Autodesk Fusion 360 part; units mm, degrees
(part 2 of 2)
sketch "Sketch6" plane through (0, 0, -2) normal (0, 0, -1) x (1, 0, 0)
  spline S0 degree 3 poles (37.9249, 4.0377) (34.348, 1.7603) (29.402, 0.3264) (25.1373, 0.3305) knots 0 0 0 0 1 1 1 1
  spline S1 degree 3 poles (25.1373, 0.3305) (25.0915, 0.3305) (25.0457, 0.3307) (25, 0.3309) knots 0 0 0 0 0.011443 0.011443 0.011443 0.011443
  spline S2 degree 3 poles (25, 0.3309) (24.9543, 0.3307) (24.9085, 0.3305) (24.8627, 0.3305) knots -0.011443 -0.011443 -0.011443 -0.011443 0 0 0 0
  spline S3 degree 3 poles (24.8627, 0.3305) (20.598, 0.3264) (15.652, 1.7603) (12.0751, 4.0377) knots -1 -1 -1 -1 0 0 0 0
  spline S4 degree 3 poles (12.0751, 4.0377) (9.8012, 5.4854) (7.8971, 7.1098) (6.2927, 8.9882) knots -1 -1 -1 -1 -0.448955 -0.448955 -0.448955 -0.448955
  spline S5 degree 5 poles (6.2927, 8.9882) (6.7312, 9.5928) (7.5942, 10.7006) (8.8467, 12.0587) (10.4463, 13.3414) (12.3768, 14.3264) (13.9094, 14.7689) (15.0688, 14.9371) (15.8476, 14.9755) (16.2364, 14.9764) knots 0 0 0 0 0 0 0.2 0.4 0.6 0.8 0.997509 0.997509 0.997509 0.997509 0.997509 0.997509
  spline S6 degree 3 poles (16.2364, 14.9764) (16.2539, 14.4812) (16.2926, 14.0359) (16.3533, 13.7321) knots 0.672801 0.672801 0.672801 0.672801 1 1 1 1
  spline S7 degree 3 poles (16.3533, 13.7321) (16.7289, 11.8523) (17.4711, 10.4695) (18.4214, 9.8792) knots 0 0 0 0 1 1 1 1
  spline S8 degree 3 poles (18.4214, 9.8792) (18.7703, 9.6625) (18.8263, 9.6487) (19.3578, 9.6487) knots 0 0 0 0 1 1 1 1
  spline S9 degree 3 poles (19.3578, 9.6487) (19.8618, 9.6487) (19.958, 9.6692) (20.2453, 9.8381) knots 0 0 0 0 1 1 1 1
  spline S10 degree 3 poles (20.2453, 9.8381) (21.4794, 10.5634) (22.3435, 12.632) (22.4858, 14.9765) knots 0 0 0 0 0.816867 0.816867 0.816867 0.816867
  line L0 (22.4858, 14.9765) -> (27.5142, 14.9765)
  spline S11 degree 3 poles (27.5142, 14.9765) (27.6565, 12.632) (28.5206, 10.5634) (29.7547, 9.8381) knots -0.816867 -0.816867 -0.816867 -0.816867 0 0 0 0
  spline S12 degree 3 poles (29.7547, 9.8381) (30.042, 9.6692) (30.1382, 9.6487) (30.6422, 9.6487) knots -1 -1 -1 -1 0 0 0 0
  spline S13 degree 3 poles (30.6422, 9.6487) (31.1737, 9.6487) (31.2297, 9.6625) (31.5786, 9.8792) knots -1 -1 -1 -1 0 0 0 0
  spline S14 degree 3 poles (31.5786, 9.8792) (32.5289, 10.4695) (33.2711, 11.8523) (33.6467, 13.7321) knots -1 -1 -1 -1 0 0 0 0
  spline S15 degree 3 poles (33.6467, 13.7321) (33.7074, 14.0359) (33.7461, 14.4812) (33.7636, 14.9764) knots -1 -1 -1 -1 -0.672801 -0.672801 -0.672801 -0.672801
  spline S16 degree 5 poles (33.7636, 14.9764) (34.1524, 14.9755) (34.9312, 14.9371) (36.0906, 14.7689) (37.6232, 14.3264) (39.5537, 13.3414) (41.1533, 12.0587) (42.4058, 10.7006) (43.2688, 9.5928) (43.7073, 8.9882) knots -0.997509 -0.997509 -0.997509 -0.997509 -0.997509 -0.997509 -0.8 -0.6 -0.4 -0.2 0 0 0 0 0 0
  spline S17 degree 3 poles (43.7073, 8.9882) (42.1029, 7.1098) (40.1988, 5.4854) (37.9249, 4.0377) knots 0.448955 0.448955 0.448955 0.448955 1 1 1 1
  line L1 (26, 42.9197) -> (26, 49.8323)
  spline S18 degree 3 poles (26, 49.8323) (26.5653, 49.8125) (27.1076, 49.7746) (27.6071, 49.7183) knots 0.743062 0.743062 0.743062 0.743062 1 1 1 1
  spline S19 degree 3 poles (27.6071, 49.7183) (31.8916, 49.2352) (35.9396, 47.6727) (39.3823, 45.1732) knots 0 0 0 0 1 1 1 1
  spline S20 degree 3 poles (39.3823, 45.1732) (40.6259, 44.2703) (41.223, 43.7559) (42.4276, 42.5496) knots 0 0 0 0 1 1 1 1
  spline S21 degree 3 poles (42.4276, 42.5496) (44.1166, 40.8584) (45.373, 39.2036) (46.5306, 37.1458) knots 0 0 0 0 1 1 1 1
  spline S22 degree 3 poles (46.5306, 37.1458) (47.3561, 35.6786) (48.2602, 33.529) (48.6498, 32.1074) knots 0 0 0 0 1 1 1 1
  spline S23 degree 3 poles (48.6498, 32.1074) (48.7491, 31.7452) (48.8843, 31.2562) (48.9503, 31.0207) knots 0 0 0 0 1 1 1 1
  spline S24 degree 3 poles (48.9503, 31.0207) (49.1719, 30.2294) (49.3568, 29.1578) (49.4818, 28.0278) knots 0 0 0 0 0.470145 0.470145 0.470145 0.470145
  spline S25 degree 3 poles (49.4818, 28.0278) (47.9315, 28.8817) (46.4271, 29.3185) (45.0223, 29.384) (43.136, 29.4719) (41.4621, 28.9779) (40.0154, 28.0751) knots 0.091067 0.091067 0.091067 0.091067 0.417024 0.417024 0.417024 0.85471 0.85471 0.85471 0.85471
  spline S26 degree 3 poles (40.0154, 28.0751) (40.0053, 28.8306) (39.9736, 29.2565) (39.904, 29.7035) knots -0.761621 -0.761621 -0.761621 -0.761621 0 0 0 0
  spline S27 degree 3 poles (39.904, 29.7035) (39.3804, 33.0647) (37.9288, 36.0367) (35.6546, 38.4035) knots -1 -1 -1 -1 0 0 0 0
  spline S28 degree 3 poles (35.6546, 38.4035) (34.8864, 39.2029) (33.7866, 40.1121) (32.9419, 40.646) knots -1 -1 -1 -1 0 0 0 0
  spline S29 degree 3 poles (32.9419, 40.646) (31.0907, 41.8162) (28.4901, 42.7183) (26.4545, 42.8964) knots -1 -1 -1 -1 0 0 0 0
  spline S30 degree 3 poles (26.4545, 42.8964) (26.3388, 42.9066) (26.1819, 42.9143) (26, 42.9197) knots -1 -1 -1 -1 -0.809548 -0.809548 -0.809548 -0.809548
  spline S31 degree 3 poles (24, 42.9197) (23.8181, 42.9143) (23.6612, 42.9066) (23.5455, 42.8964) knots 0.809548 0.809548 0.809548 0.809548 1 1 1 1
  spline S32 degree 3 poles (23.5455, 42.8964) (21.5099, 42.7183) (18.9093, 41.8162) (17.0581, 40.646) knots 0 0 0 0 1 1 1 1
  spline S33 degree 3 poles (17.0581, 40.646) (16.2134, 40.1121) (15.1136, 39.2029) (14.3454, 38.4035) knots 0 0 0 0 1 1 1 1
  spline S34 degree 3 poles (14.3454, 38.4035) (12.0712, 36.0367) (10.6196, 33.0647) (10.096, 29.7035) knots 0 0 0 0 1 1 1 1
  spline S35 degree 3 poles (10.096, 29.7035) (10.0264, 29.2565) (9.9947, 28.8306) (9.9846, 28.0751) knots 0 0 0 0 0.761621 0.761621 0.761621 0.761621
  spline S36 degree 3 poles (9.9846, 28.0751) (8.5379, 28.9779) (6.864, 29.4719) (4.9777, 29.384) (3.5729, 29.3185) (2.0685, 28.8817) (0.5182, 28.0278) knots -0.85471 -0.85471 -0.85471 -0.85471 -0.417024 -0.417024 -0.417024 -0.091067 -0.091067 -0.091067 -0.091067
  spline S37 degree 3 poles (0.5182, 28.0278) (0.6432, 29.1578) (0.8281, 30.2294) (1.0497, 31.0207) knots -0.470145 -0.470145 -0.470145 -0.470145 0 0 0 0
  spline S38 degree 3 poles (1.0497, 31.0207) (1.1157, 31.2562) (1.2509, 31.7452) (1.3502, 32.1074) knots -1 -1 -1 -1 0 0 0 0
  spline S39 degree 3 poles (1.3502, 32.1074) (1.7398, 33.529) (2.6439, 35.6786) (3.4694, 37.1458) knots -1 -1 -1 -1 0 0 0 0
  spline S40 degree 3 poles (3.4694, 37.1458) (4.627, 39.2036) (5.8834, 40.8584) (7.5724, 42.5496) knots -1 -1 -1 -1 0 0 0 0
  spline S41 degree 3 poles (7.5724, 42.5496) (8.777, 43.7559) (9.3741, 44.2703) (10.6177, 45.1732) knots -1 -1 -1 -1 0 0 0 0
  spline S42 degree 3 poles (10.6177, 45.1732) (14.0604, 47.6727) (18.1084, 49.2352) (22.3929, 49.7183) knots -1 -1 -1 -1 0 0 0 0
  spline S43 degree 3 poles (22.3929, 49.7183) (22.8924, 49.7746) (23.4347, 49.8125) (24, 49.8323) knots -1 -1 -1 -1 -0.743062 -0.743062 -0.743062 -0.743062
  line L2 (24, 49.8323) -> (24, 42.9197)
  spline S44 degree 3 poles (49.6438, 24.3029) (49.4952, 20.5588) (48.6987, 17.4096) (47.0703, 14.1273) knots 0 0 0 0 1 1 1 1
  spline S45 degree 3 poles (47.0703, 14.1273) (46.493, 12.9638) (45.8561, 11.8785) (45.1508, 10.8618) knots 0 0 0 0 0.273539 0.273539 0.273539 0.273539
  spline S46 degree 3 poles (45.1508, 10.8618) (43.4717, 13.1181) (41.7533, 14.5837) (40.0547, 15.4812) (38.2296, 16.4456) (36.4871, 16.8223) (34.777, 16.9413) (34.4324, 16.9653) (34.0883, 16.9769) (33.7445, 16.9765) (33.738, 16.9765) (33.7315, 16.9765) (33.725, 16.9765) knots 0.013228 0.013228 0.013228 0.013228 0.443948 0.443948 0.443948 0.906729 0.906729 0.906729 1 1 1 1.00195 1.00195 1.00195 1.00195
  ellipse E0 centre (33.3549, 15.0887) end of major axis (33.411, 18.2873) minor radius 0.4181 (33.725, 16.9765) -> (33.6101, 17.8664) ccw
  spline S47 degree 3 poles (33.6101, 17.8664) (33.169, 19.9501) (32.2562, 21.4052) (31.1636, 21.7662) knots -1 -1 -1 -1 0 0 0 0
  spline S48 degree 3 poles (31.1636, 21.7662) (30.3753, 22.0267) (29.4073, 21.5865) (28.8005, 20.6915) knots -1 -1 -1 -1 0 0 0 0
  spline S49 degree 3 poles (28.8005, 20.6915) (28.1198, 19.6876) (27.7379, 18.5421) (27.5687, 16.9765) knots -1 -1 -1 -1 -0.075763 -0.075763 -0.075763 -0.075763
  line L3 (27.5687, 16.9765) -> (22.4313, 16.9765)
  spline S50 degree 3 poles (22.4313, 16.9765) (22.2621, 18.5421) (21.8802, 19.6876) (21.1995, 20.6915) knots 0.075763 0.075763 0.075763 0.075763 1 1 1 1
  spline S51 degree 3 poles (21.1995, 20.6915) (20.5927, 21.5865) (19.6247, 22.0267) (18.8364, 21.7662) knots 0 0 0 0 1 1 1 1
  spline S52 degree 3 poles (18.8364, 21.7662) (17.7438, 21.4052) (16.831, 19.9501) (16.3899, 17.8664) knots 0 0 0 0 1 1 1 1
  ellipse E1 centre (16.6451, 15.0887) end of major axis (16.7011, 11.8901) minor radius 0.4181 (16.3899, 17.8664) -> (16.275, 16.9765) ccw
  spline S53 degree 3 poles (16.275, 16.9765) (16.2685, 16.9765) (16.262, 16.9765) (16.2555, 16.9765) (15.9117, 16.9769) (15.5676, 16.9653) (15.223, 16.9413) (13.5129, 16.8223) (11.7704, 16.4456) (9.9453, 15.4812) (8.2467, 14.5837) (6.5283, 13.1181) (4.8492, 10.8618) knots -1.00195 -1.00195 -1.00195 -1.00195 -1 -1 -1 -0.906729 -0.906729 -0.906729 -0.443948 -0.443948 -0.443948 -0.013228 -0.013228 -0.013228 -0.013228
  spline S54 degree 3 poles (4.8492, 10.8618) (4.1439, 11.8785) (3.507, 12.9638) (2.9297, 14.1273) knots -0.273539 -0.273539 -0.273539 -0.273539 0 0 0 0
  spline S55 degree 3 poles (2.9297, 14.1273) (1.3013, 17.4096) (0.5048, 20.5588) (0.3562, 24.3029) knots -1 -1 -1 -1 0 0 0 0
  ellipse E2 centre (1.5341, 27.8391) end of major axis (0.9284, 22.1103) minor radius 1.0317 (0.3495, 25.5702) -> (0.3562, 24.3029) ccw
  spline S56 degree 5 poles (0.3495, 25.5702) (0.8642, 25.9274) (1.8614, 26.5452) (3.261, 27.1829) (4.9563, 27.5281) (6.8533, 27.3542) (8.214, 26.8513) (9.1392, 26.2868) (9.7099, 25.8236) (9.9837, 25.5702) knots 0 0 0 0 0 0 0.2 0.4 0.6 0.8 1 1 1 1 1 1
  line L4 (9.9837, 25.5702) -> (9.5685, 25.3593)
  spline S57 degree 3 poles (9.5685, 25.3593) (8.985, 25.0629) (8.7925, 24.7926) (8.7925, 24.2699) knots 0 0 0 0 1 1 1 1
  spline S58 degree 3 poles (8.7925, 24.2699) (8.7925, 23.9246) (8.8206, 23.8276) (8.9823, 23.6157) knots 0 0 0 0 1 1 1 1
  spline S59 degree 3 poles (8.9823, 23.6157) (9.0867, 23.4788) (9.271, 23.3255) (9.3918, 23.275) knots 0 0 0 0 1 1 1 1
  spline S60 degree 3 poles (9.3918, 23.275) (9.865, 23.0773) (10.0223, 23.1273) (11.92, 24.0791) knots 0 0 0 0 1 1 1 1
  spline S61 degree 3 poles (11.92, 24.0791) (13.4801, 24.8616) (13.727, 25.0063) (13.87, 25.2225) knots 0 0 0 0 1 1 1 1
  spline S62 degree 3 poles (13.87, 25.2225) (14.3541, 25.9539) (13.9374, 26.8519) (13.081, 26.923) knots 0 0 0 0 1 1 1 1
  spline S63 degree 3 poles (13.081, 26.923) (12.7923, 26.9469) (12.6703, 26.9186) (12.3363, 26.7499) knots 0 0 0 0 1 1 1 1
  ellipse E3 centre (12.2838, 26.7829) end of major axis (12.6728, 26.975) minor radius 0.053 (11.8959, 26.5891) -> (12.3363, 26.7499) ccw
  spline S64 degree 3 poles (11.8959, 26.5891) (11.7452, 26.7398) (11.9635, 29.5037) (12.2147, 30.6256) knots 0 0 0 0 1 1 1 1
  spline S65 degree 3 poles (12.2147, 30.6256) (12.3647, 31.2958) (12.9496, 32.9532) (13.2453, 33.5457) knots 0 0 0 0 1 1 1 1
  spline S66 degree 3 poles (13.2453, 33.5457) (14.0979, 35.2549) (15.1952, 36.6806) (16.5766, 37.8744) knots 0 0 0 0 1 1 1 1
  spline S67 degree 3 poles (16.5766, 37.8744) (18.9879, 39.9581) (21.902, 41.0359) (25, 41.0162) knots 0 0 0 0 0.826651 0.826651 0.826651 0.826651
  spline S68 degree 3 poles (25, 41.0162) (28.098, 41.0359) (31.0121, 39.9581) (33.4234, 37.8744) knots -0.826651 -0.826651 -0.826651 -0.826651 0 0 0 0
  spline S69 degree 3 poles (33.4234, 37.8744) (34.8048, 36.6806) (35.9021, 35.2549) (36.7547, 33.5457) knots -1 -1 -1 -1 0 0 0 0
  spline S70 degree 3 poles (36.7547, 33.5457) (37.0504, 32.9532) (37.6353, 31.2958) (37.7853, 30.6256) knots -1 -1 -1 -1 0 0 0 0
  spline S71 degree 3 poles (37.7853, 30.6256) (38.0365, 29.5037) (38.2548, 26.7398) (38.1041, 26.5891) knots -1 -1 -1 -1 0 0 0 0
  ellipse E4 centre (37.7162, 26.7829) end of major axis (38.1053, 26.5908) minor radius 0.053 (37.6637, 26.7499) -> (38.1041, 26.5891) ccw
  spline S72 degree 3 poles (37.6637, 26.7499) (37.3297, 26.9186) (37.2077, 26.9469) (36.919, 26.923) knots -1 -1 -1 -1 0 0 0 0
  spline S73 degree 3 poles (36.919, 26.923) (36.0626, 26.8519) (35.6459, 25.9539) (36.13, 25.2225) knots -1 -1 -1 -1 0 0 0 0
  spline S74 degree 3 poles (36.13, 25.2225) (36.273, 25.0063) (36.5199, 24.8616) (38.08, 24.0791) knots -1 -1 -1 -1 0 0 0 0
  spline S75 degree 3 poles (38.08, 24.0791) (39.9777, 23.1273) (40.135, 23.0773) (40.6082, 23.275) knots -1 -1 -1 -1 0 0 0 0
  spline S76 degree 3 poles (40.6082, 23.275) (40.729, 23.3255) (40.9133, 23.4788) (41.0177, 23.6157) knots -1 -1 -1 -1 0 0 0 0
  spline S77 degree 3 poles (41.0177, 23.6157) (41.1794, 23.8276) (41.2075, 23.9246) (41.2075, 24.2699) knots -1 -1 -1 -1 0 0 0 0
  spline S78 degree 3 poles (41.2075, 24.2699) (41.2075, 24.7926) (41.015, 25.0629) (40.4315, 25.3593) knots -1 -1 -1 -1 0 0 0 0
  line L5 (40.4315, 25.3593) -> (40.0163, 25.5702)
  spline S79 degree 5 poles (40.0163, 25.5702) (40.2901, 25.8236) (40.8608, 26.2868) (41.786, 26.8513) (43.1467, 27.3542) (45.0437, 27.5281) (46.739, 27.1829) (48.1386, 26.5452) (49.1358, 25.9274) (49.6505, 25.5702) knots -1 -1 -1 -1 -1 -1 -0.8 -0.6 -0.4 -0.2 0 0 0 0 0 0
  ellipse E5 centre (48.4659, 27.8391) end of major axis (47.8603, 33.5679) minor radius 1.0317 (49.6438, 24.3029) -> (49.6505, 25.5702) ccw
  spline S80 degree 3 poles (27.7416, 50.9107) (26.8953, 51.0062) (25.9601, 51.0501) (24.9982, 51.0487) knots -1 -1 -1 -1 -0.594454 -0.594454 -0.594454 -0.594454
  spline S81 degree 3 poles (24.9982, 51.0487) (24.0376, 51.05) (23.1037, 51.006) (22.2584, 50.9107) knots 0.594956 0.594956 0.594956 0.594956 1 1 1 1
  spline S82 degree 3 poles (22.2584, 50.9107) (17.7713, 50.4048) (13.5248, 48.7669) (9.9127, 46.1443) knots 0 0 0 0 1 1 1 1
  spline S83 degree 3 poles (9.9127, 46.1443) (8.6415, 45.2214) (7.9474, 44.6234) (6.7233, 43.3976) knots 0 0 0 0 1 1 1 1
  spline S84 degree 3 poles (6.7233, 43.3976) (4.968, 41.64) (3.6282, 39.8758) (2.4235, 37.7342) knots 0 0 0 0 1 1 1 1
  spline S85 degree 3 poles (2.4235, 37.7342) (1.5361, 36.1568) (0.6261, 34.0052) (0.1929, 32.4246) knots 0 0 0 0 1 1 1 1
  spline S86 degree 3 poles (0.1929, 32.4246) (0.0942, 32.0647) (-0.0413, 31.5745) (-0.1058, 31.3445) knots 0 0 0 0 0.999998 0.999998 0.999998 0.999998
  spline S87 degree 3 poles (-0.1058, 31.3445) (-0.5059, 29.9163) (-0.7593, 27.9125) (-0.8356, 26.045) (-0.861, 25.4219) (-0.8652, 24.8169) (-0.8429, 24.2553) knots 0 0 0 0 0.749811 0.749811 0.749811 1 1 1 1
  spline S88 degree 3 poles (-0.8429, 24.2553) (-0.6886, 20.3681) (0.1597, 17.0105) (1.8548, 13.5939) knots 0 0 0 0 1 1 1 1
  spline S89 degree 3 poles (1.8548, 13.5939) (4.0534, 9.1625) (7.1462, 5.7533) (11.4307, 3.0254) knots 0 0 0 0 1 1 1 1
  spline S90 degree 3 poles (11.4307, 3.0254) (15.2378, 0.6015) (20.3293, -0.8738) (24.8638, -0.8695) knots 0 0 0 0 1 1 1 1
  spline S91 degree 3 poles (24.8638, -0.8695) (24.9093, -0.8695) (24.9547, -0.8693) (25, -0.8691) knots 0 0 0 0 0.010916 0.010916 0.010916 0.010916
  spline S92 degree 3 poles (25, -0.8691) (25.0453, -0.8693) (25.0907, -0.8695) (25.1362, -0.8695) knots -0.010916 -0.010916 -0.010916 -0.010916 0 0 0 0
  spline S93 degree 3 poles (25.1362, -0.8695) (29.6707, -0.8738) (34.7622, 0.6015) (38.5693, 3.0254) knots -1 -1 -1 -1 0 0 0 0
  spline S94 degree 3 poles (38.5693, 3.0254) (42.8538, 5.7533) (45.9466, 9.1625) (48.1452, 13.5939) knots -1 -1 -1 -1 0 0 0 0
  spline S95 degree 3 poles (48.1452, 13.5939) (49.8403, 17.0105) (50.6886, 20.3681) (50.8429, 24.2553) knots -1 -1 -1 -1 0 0 0 0
  spline S96 degree 3 poles (50.8429, 24.2553) (50.8652, 24.8169) (50.861, 25.4219) (50.8356, 26.045) (50.7593, 27.9125) (50.5059, 29.9163) (50.1058, 31.3445) knots -1 -1 -1 -1 -0.749811 -0.749811 -0.749811 0 0 0 0
  spline S97 degree 3 poles (50.1058, 31.3445) (50.0413, 31.5744) (49.9058, 32.0647) (49.8071, 32.4246) knots -1 -1 -1 -1 0 0 0 0
  spline S98 degree 3 poles (49.8071, 32.4246) (49.3739, 34.0052) (48.4639, 36.1568) (47.5765, 37.7342) knots -1 -1 -1 -1 0 0 0 0
  spline S99 degree 3 poles (47.5765, 37.7342) (46.3718, 39.8758) (45.032, 41.64) (43.2767, 43.3976) knots -1 -1 -1 -1 0 0 0 0
  spline S100 degree 3 poles (43.2767, 43.3976) (42.0526, 44.6234) (41.3585, 45.2214) (40.0873, 46.1443) knots -1 -1 -1 -1 0 0 0 0
  spline S101 degree 3 poles (40.0873, 46.1443) (36.4752, 48.7669) (32.2287, 50.4048) (27.7416, 50.9107) knots -1 -1 -1 -1 0 0 0 0
  spline S102 degree 3 poles (53.3409, 24.1561) (53.3665, 24.8011) (53.3612, 25.469) (53.3335, 26.1471) (53.2588, 27.977) (53.0414, 29.8835) (52.6441, 31.5169) (52.6028, 31.6868) (52.5592, 31.8541) (52.5131, 32.0189) knots -1 -1 -1 -1 -0.749811 -0.749811 -0.749811 -0.07064 -0.07064 -0.07064 0 0 0 0
  spline S103 degree 3 poles (52.5131, 32.0189) (52.4519, 32.2373) (52.3155, 32.7305) (52.2182, 33.0855) knots -0.999997 -0.999997 -0.999997 -0.999997 0 0 0 0
  spline S104 degree 3 poles (52.2182, 33.0855) (51.7442, 34.8149) (50.9078, 36.812) (50.0002, 38.513) (49.9193, 38.6646) (49.8377, 38.8137) (49.7554, 38.9599) knots -1 -1 -1 -1 -0.081824 -0.081824 -0.081824 0 0 0 0
  spline S105 degree 3 poles (49.7554, 38.9599) (48.45, 41.2805) (46.9425, 43.2648) (45.0457, 45.1642) knots -1 -1 -1 -1 0 0 0 0
  spline S106 degree 3 poles (45.0457, 45.1642) (43.7749, 46.4367) (42.8926, 47.197) (41.5561, 48.1673) knots -1 -1 -1 -1 0 0 0 0
  spline S107 degree 3 poles (41.5561, 48.1673) (37.5906, 51.0464) (32.9313, 52.8415) (28.0217, 53.395) knots -1 -1 -1 -1 0 0 0 0
  spline S108 degree 3 poles (28.0217, 53.395) (27.0588, 53.5036) (26.0396, 53.55) (25.0016, 53.5487) knots -1 -1 -1 -1 -0.595383 -0.595383 -0.595383 -0.595383
  spline S109 degree 3 poles (25.0016, 53.5487) (23.9625, 53.5501) (22.9423, 53.5037) (21.9783, 53.395) knots 0.594956 0.594956 0.594956 0.594956 1 1 1 1
  spline S110 degree 3 poles (21.9783, 53.395) (17.0687, 52.8415) (12.4094, 51.0464) (8.4439, 48.1673) knots 0 0 0 0 1 1 1 1
  spline S111 degree 3 poles (8.4439, 48.1673) (7.1074, 47.197) (6.2251, 46.4367) (4.9543, 45.1642) knots 0 0 0 0 1 1 1 1
  spline S112 degree 3 poles (4.9543, 45.1642) (3.0575, 43.2648) (1.55, 41.2805) (0.2446, 38.9599) knots 0 0 0 0 1 1 1 1
  spline S113 degree 3 poles (0.2446, 38.9599) (-0.6787, 37.3187) (-1.5454, 35.3158) (-2.0829, 33.5523) (-2.1308, 33.3952) (-2.176, 33.2396) (-2.2182, 33.0855) knots 0 0 0 0 0.918176 0.918176 0.918176 1 1 1 1
  spline S114 degree 3 poles (-2.2182, 33.0855) (-2.3155, 32.7305) (-2.4519, 32.2373) (-2.5131, 32.0189) knots 0 0 0 0 0.999998 0.999998 0.999998 0.999998
  spline S115 degree 3 poles (-2.5131, 32.0189) (-2.9569, 30.4347) (-3.1982, 28.5652) (-3.3052, 26.7206) (-3.3163, 26.5287) (-3.3257, 26.3374) (-3.3335, 26.1471) (-3.3612, 25.469) (-3.3665, 24.8011) (-3.3409, 24.1561) knots 0 0 0 0 0.679172 0.679172 0.679172 0.749811 0.749811 0.749811 1 1 1 1
  spline S116 degree 3 poles (-3.3409, 24.1561) (-3.1745, 19.9631) (-2.2221, 16.1861) (-0.3848, 12.4828) knots 0 0 0 0 1 1 1 1
  spline S117 degree 3 poles (-0.3848, 12.4828) (2.0018, 7.6725) (5.4673, 3.8585) (10.088, 0.9166) knots 0 0 0 0 1 1 1 1
  spline S118 degree 3 poles (10.088, 0.9166) (13.6936, -1.3791) (18.1285, -2.8408) (22.4732, -3.2545) (23.2753, -3.3308) (24.0747, -3.3703) (24.8662, -3.3695) knots 0 0 0 0 0.844152 0.844152 0.844152 1 1 1 1
  spline S119 degree 3 poles (24.8662, -3.3695) (24.9108, -3.3695) (24.9554, -3.3694) (25, -3.3691) knots 0 0 0 0 0.009937 0.009937 0.009937 0.009937
  spline S120 degree 3 poles (25, -3.3691) (25.0446, -3.3694) (25.0892, -3.3695) (25.1338, -3.3695) knots -0.009937 -0.009937 -0.009937 -0.009937 0 0 0 0
  spline S121 degree 3 poles (25.1338, -3.3695) (29.4209, -3.3736) (33.9529, -2.2384) (37.8353, -0.2655) (38.552, 0.0987) (39.2463, 0.4927) (39.912, 0.9166) knots -1 -1 -1 -1 -0.155848 -0.155848 -0.155848 0 0 0 0
  spline S122 degree 3 poles (39.912, 0.9166) (44.5327, 3.8585) (47.9982, 7.6725) (50.3848, 12.4828) knots -1 -1 -1 -1 0 0 0 0
  spline S123 degree 3 poles (50.3848, 12.4828) (52.222, 16.1861) (53.1745, 19.9631) (53.3409, 24.1561) knots -1 -1 -1 -1 0 0 0 0
  spline S124 degree 3 poles (48.3448, 24.3544) (48.3638, 24.8327) (48.3609, 25.3748) (48.3377, 25.943) (48.2742, 27.4962) (48.0627, 29.1964) (47.7857, 30.3352) (47.7569, 30.4537) (47.7277, 30.5657) (47.6984, 30.67) knots -1 -1 -1 -1 -0.749811 -0.749811 -0.749811 -0.07064 -0.07064 -0.07064 0 0 0 0
  spline S125 degree 3 poles (47.6984, 30.67) (47.6308, 30.9116) (47.496, 31.399) (47.396, 31.7638) knots -1 -1 -1 -1 0 0 0 0
  spline S126 degree 3 poles (47.396, 31.7638) (47.0745, 32.9368) (46.3114, 34.8051) (45.5889, 36.1592) (45.5245, 36.2798) (45.4606, 36.3966) (45.3976, 36.5085) knots -1 -1 -1 -1 -0.081824 -0.081824 -0.081824 0 0 0 0
  spline S127 degree 3 poles (45.3976, 36.5085) (44.2935, 38.4711) (43.1214, 40.0152) (41.5078, 41.631) knots -1 -1 -1 -1 0 0 0 0
  spline S128 degree 3 poles (41.5078, 41.631) (40.3302, 42.8101) (39.8244, 43.2458) (38.6185, 44.1213) knots -1 -1 -1 -1 0 0 0 0
  spline S129 degree 3 poles (38.6185, 44.1213) (35.3597, 46.4873) (31.5261, 47.9682) (27.4615, 48.4265) knots -1 -1 -1 -1 0 0 0 0
  spline S130 degree 3 poles (27.4615, 48.4265) (26.734, 48.5085) (25.8853, 48.55) (25.0019, 48.5487) (25.0013, 48.5487) (25.0007, 48.5487) (25.0001, 48.5487) knots -1 -1 -1 -1 -0.594454 -0.594454 -0.594454 -0.594202 -0.594202 -0.594202 -0.594202
  spline S131 degree 3 poles (25.0001, 48.5487) (24.9984, 48.5487) (24.9966, 48.5487) (24.9948, 48.5487) (24.1126, 48.5499) (23.2651, 48.5084) (22.5385, 48.4265) knots 0.594203 0.594203 0.594203 0.594203 0.594956 0.594956 0.594956 1 1 1 1
  spline S132 degree 3 poles (22.5385, 48.4265) (18.4739, 47.9682) (14.6403, 46.4873) (11.3815, 44.1213) knots 0 0 0 0 1 1 1 1
  spline S133 degree 3 poles (11.3815, 44.1213) (10.1756, 43.2458) (9.6698, 42.8101) (8.4922, 41.631) knots 0 0 0 0 1 1 1 1
  spline S134 degree 3 poles (8.4922, 41.631) (6.8786, 40.0152) (5.7065, 38.4711) (4.6024, 36.5085) knots 0 0 0 0 1 1 1 1
  spline S135 degree 3 poles (4.6024, 36.5085) (3.8961, 35.253) (3.0951, 33.3911) (2.6999, 32.0946) (2.6647, 31.979) (2.6326, 31.8683) (2.604, 31.7638) knots 0 0 0 0 0.918176 0.918176 0.918176 1 1 1 1
  spline S136 degree 3 poles (2.604, 31.7638) (2.504, 31.399) (2.3692, 30.9116) (2.3016, 30.67) knots 0 0 0 0 0.999998 0.999998 0.999998 0.999998
  spline S137 degree 3 poles (2.3015, 30.67) (2.0206, 29.667) (1.7777, 28.0047) (1.6865, 26.4312) (1.677, 26.2675) (1.6689, 26.1046) (1.6623, 25.943) (1.6391, 25.3748) (1.6362, 24.8327) (1.6552, 24.3544) knots 0 0 0 0 0.679172 0.679172 0.679172 0.749811 0.749811 0.749811 1 1 1 1
  spline S138 degree 3 poles (1.6552, 24.3544) (1.7973, 20.7731) (2.5415, 17.8349) (4.0943, 14.705) knots 0 0 0 0 1 1 1 1
  spline S139 degree 3 poles (4.0943, 14.705) (6.1049, 10.6525) (8.8251, 7.648) (12.7733, 5.1343) knots 0 0 0 0 1 1 1 1
  spline S140 degree 3 poles (12.7733, 5.1343) (15.5953, 3.3375) (19.4185, 2.059) (22.9471, 1.723) (23.5985, 1.661) (24.2395, 1.6299) (24.8615, 1.6305) knots 0 0 0 0 0.844152 0.844152 0.844152 1 1 1 1
  spline S141 degree 3 poles (24.8615, 1.6305) (24.9033, 1.6305) (24.9451, 1.6306) (24.9868, 1.6309) (24.9912, 1.6309) (24.9956, 1.6309) (25, 1.6309) knots 0 0 0 0 0.010916 0.010916 0.010916 0.011972 0.011972 0.011972 0.011972
  spline S142 degree 3 poles (25, 1.6309) (25.0044, 1.6309) (25.0088, 1.6309) (25.0132, 1.6309) (25.0549, 1.6306) (25.0967, 1.6305) (25.1385, 1.6305) knots -0.011972 -0.011972 -0.011972 -0.011972 -0.010916 -0.010916 -0.010916 0 0 0 0
  spline S143 degree 3 poles (25.1385, 1.6305) (28.5072, 1.6273) (32.4245, 2.5935) (35.5702, 4.192) (36.1509, 4.4871) (36.7057, 4.8025) (37.2267, 5.1343) knots -1 -1 -1 -1 -0.155848 -0.155848 -0.155848 0 0 0 0
  spline S144 degree 3 poles (37.2267, 5.1343) (41.1749, 7.648) (43.8951, 10.6525) (45.9057, 14.705) knots -1 -1 -1 -1 0 0 0 0
  spline S145 degree 3 poles (45.9057, 14.705) (47.4585, 17.8349) (48.2027, 20.7731) (48.3448, 24.3544) knots -1 -1 -1 -1 0 0 0 0
  dimension "d20" = 2.5
  dimension "d21" = -2.5
extrude "Extrude4" add sketch "Sketch6" against normal up to surface (2 mm away) contours S0 S1 S2 S3 S4 S5 S16 S17 S139 S140 S141 S142 S143 S144 | S44 S45 S46 S79 E5 S124 S144 S145 | S53 S54 S55 E2 S56 S137 S138 S139 | L1 S18 S19 S20 S21 S22 S23 S24 S25 S124 S125 S126 S127 S128 S129 S130 | S36 S37 S38 S39 S40 S41 S42 S43 L2 S131 S132 S133 S134 S135 S136 S137
equation "CuttingHeight = 10 mm"
equation "IndentHeight = 5 mm"
equation "FlangeWidth = 2 mm"
equation "CutterWidth = 1.2 mm"
equation "FlangeThickness = 2 mm"
equation "d9 = CutterWidth"
equation "d14 = -FlangeThickness"
equation "d16 = CuttingHeight"
equation "d18 = IndentHeight"
